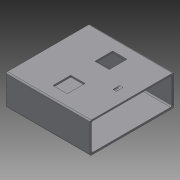
# Autodesk Inventor part: USB-Connector1
Saved by Autodesk Inventor 2015 (Build 190159000, 159)
## iProperties
Created: 2021-05-12
Part Number: USB-Connector1
Material: Generic
Document SubType Name: Modeling
Designer: bayua
Density: 1 g/cm^3
Appearance: Default
Author: bayua
Autodesk Inventor part; units mm, degrees
ref_plane "YZ Plane" through (0, 0, 0) normal (1, 0, 0) x (0, 1, 0)
ref_plane "XZ Plane" through (0, 0, 0) normal (0, 1, 0) x (-1, 0, 0)
ref_plane "XY Plane" through (0, 0, 0) normal (0, 0, 1) x (1, 0, 0)
sketch "Sketch2" plane through (0, 0, 0) normal (0, 0, 1) x (1, 0, 0)
  line L0 (-6.096, 6.096) -> (6.096, 6.096)
  line L1 (6.096, 6.096) -> (6.096, -6.096)
  line L2 (6.096, -6.096) -> (-6.096, -6.096)
  line L3 (-6.096, -6.096) -> (-6.096, 6.096)
  point P0 (0, 0)
  dimension "d4" = 12.192
  dimension "d5" = 12.192
  dimension "d6" = 6.096
  dimension "d7" = 6.096
  constraints: 8 end point, 2 parallel, 1 horizontal, 1 perpendicular
  measures "d4" distance of L0.end L1.end
  measures "d5" distance of L1.end L2.end
  measures "d6" distance from line of point (0, 0) L1
  measures "d7" distance from line of point (0, 0) L0
extrude "Extrusion1" add sketch "Sketch2" along normal mid plane 4.445
sketch "Sketch3" plane through (6.096, -6.096, 2.2225) normal (1, 0, 0) x (0, 0, -1)
  line L0 (0.254, 11.938) -> (4.191, 11.938)
  line L1 (4.191, 11.938) -> (4.191, 0.254)
  line L2 (4.191, 0.254) -> (0.254, 0.254)
  line L3 (0.254, 0.254) -> (0.254, 11.938)
  line L4 (0, 12.192) -> (0, 0) projected
  line L5 (4.445, 12.192) -> (0, 12.192) projected
  line L6 (4.445, 12.192) -> (4.445, 0) projected
  line L7 (0, 0) -> (4.445, 0) projected
  point P0 (2.2225, 6.096)
  dimension "d10" = 0.254
  dimension "d11" = 0.254
  dimension "d12" = 0.254
  dimension "d13" = 0.254
  constraints: 8 end point, 2 parallel, 1 horizontal, 1 perpendicular
  measures "d10" distance between parallel lines of L4 L3
  measures "d11" distance between parallel lines of L5 L0
  measures "d12" distance between parallel lines of L6 L1
  measures "d13" distance between parallel lines of L7 L2
extrude "Extrusion2" cut sketch "Sketch3" against normal through all contours L0 L1 L2 L3
sketch "Sketch4" plane through (0, 0, 2.2225) normal (0, 0, 1) x (1, 0, 0)
  line L0 (-1.016, 4.318) -> (1.016, 4.318)
  line L1 (1.016, 4.318) -> (1.016, 1.778)
  line L2 (1.016, 1.778) -> (-1.016, 1.778)
  line L3 (-1.016, 1.778) -> (-1.016, 4.318)
  line L4 (6.096, -6.096) -> (6.096, 6.096) projected
  line L5 (6.096, 6.096) -> (-6.096, 6.096) projected
  point P0 (0, 0)
  dimension "d16" = 5.08
  dimension "d17" = 1.778
  dimension "d18" = 2.54
  dimension "d19" = 2.032
  constraints: 8 end point, 2 parallel, 1 horizontal, 1 perpendicular
  measures "d16" distance between parallel lines of L4 L1
  measures "d17" distance between parallel lines of L5 L0
  measures "d18" distance of L0.end L1.end
  measures "d19" distance of L0.start L0.end
extrude "Extrusion3" cut sketch "Sketch4" against normal through all
mirror "Mirror1" about plane through (0, 0, 0) normal (0, 1, 0) of "Extrusion3"
sketch "Sketch5" plane through (0, 0, -2.2225) normal (0, 0, -1) x (-1, 0, 0)
  line L0 (-6.096, -6.096) -> (-6.096, 6.096) projected
  line L1 (6.096, 5.842) -> (6.096, -5.842) projected
  line L2 (-6.096, 0.0762) -> (6.096, 0.0762)
  line L3 (6.096, 0.0762) -> (6.096, -0.0762)
  line L4 (-6.096, -0.0762) -> (-6.096, 0.0762)
  line L5 (4.5615, -0.0961) -> (4.7095, -0.3103)
  line L6 (4.699, -0.3302) -> (4.318, -0.3302)
  line L7 (4.318, -0.3302) -> (4.318, -0.0762)
  line L8 (6.096, -0.0762) -> (4.572, -0.0762)
  arc A0 (4.572, -0.0762) -> (4.5615, -0.0961) centre (4.572, -0.0889) ccw
  arc A1 (4.699, -0.3302) -> (4.7095, -0.3103) centre (4.699, -0.3175) ccw
  line L9 (4.0745, -0.0961) -> (3.9265, -0.3103)
  line L10 (3.937, -0.3302) -> (4.318, -0.3302)
  arc A2 (4.0745, -0.0961) -> (4.064, -0.0762) centre (4.064, -0.0889) ccw
  arc A3 (3.9265, -0.3103) -> (3.937, -0.3302) centre (3.937, -0.3175) ccw
  line L11 (-4.5615, -0.0961) -> (-4.7095, -0.3103)
  line L12 (-4.699, -0.3302) -> (-4.318, -0.3302)
  arc A4 (-4.5615, -0.0961) -> (-4.572, -0.0762) centre (-4.572, -0.0889) ccw
  arc A5 (-4.7095, -0.3103) -> (-4.699, -0.3302) centre (-4.699, -0.3175) ccw
  arc A6 (-4.064, -0.0762) -> (-4.0745, -0.0961) centre (-4.064, -0.0889) ccw
  line L13 (-4.0745, -0.0961) -> (-3.9265, -0.3103)
  arc A7 (-3.937, -0.3302) -> (-3.9265, -0.3103) centre (-3.937, -0.3175) ccw
  line L14 (-3.937, -0.3302) -> (-4.318, -0.3302)
  line L15 (4.064, -0.0762) -> (-4.064, -0.0762)
  line L16 (-4.572, -0.0762) -> (-6.096, -0.0762)
  point P0 (0, 0)
  dimension "d22" = 0.0762
  dimension "d25" = 0.0762
  dimension "d26" = 0.254
  dimension "d27" = 0.0127
  dimension "d28" = 1.524
  dimension "d29" = 1.397
  dimension "d30" = 1.778
  constraints: 30 end point, 16 point on circle, 8 centre point, 6 symmetric about line, 4 tangent, 2 horizontal, 2 parallel, 2 perpendicular, 2 point on line, 1 equal radius, 2 other
  measures "d22" distance from line of point (0, 0) L2
  measures "d25" distance from line of point (0, 0) L8
  measures "d26" distance between parallel lines of L8 L6
  measures "d27" radius of A0
  measures "d28" distance from line of L1 A0.centre
  measures "d29" distance from line of L1 A1.centre
  measures "d30" distance from line of L1 L7.end
extrude "Extrusion4" add sketch "Sketch5" along normal blind 0.0032
sketch "Sketch6" plane through (0, 0, 2.2225) normal (0, 0, 1) x (1, 0, 0)
  line L0 (3.81, 0.508) -> (4.318, 0.508)
  line L1 (4.318, 0.508) -> (4.318, -0.508)
  line L2 (4.318, -0.508) -> (3.81, -0.508)
  line L3 (3.81, -0.508) -> (3.81, 0.508)
  line L4 (6.096, 6.096) -> (-6.096, 6.096) projected
  line L5 (6.096, -6.096) -> (6.096, 6.096) projected
  point P0 (0, 0)
  dimension "d33" = 5.588
  dimension "d34" = 1.778
  dimension "d35" = 0.508
  dimension "d36" = 1.016
  constraints: 8 end point, 2 parallel, 1 horizontal, 1 perpendicular
  measures "d33" distance between parallel lines of L4 L0
  measures "d34" distance between parallel lines of L5 L1
  measures "d35" distance of L0.start L0.end
  measures "d36" distance of L0.end L1.end
extrude "Extrusion5" cut sketch "Sketch6" against normal blind 0.127
fillet "Fillet1" radius 0.635 2 edges at (4.064, 0.508, 2.0955) (4.064, -0.508, 2.0955)
fillet "Fillet2" radius 0.0635 6 edges at (3.81, 0.3278, 2.1281) (3.81, -0.3278, 2.1281) (3.81, 0, 2.0955) (4.318, -0.3278, 2.1281) (4.318, 0.3278, 2.1281) (4.318, 0, 2.0955)
fillet "Fillet3" radius 0.1905 8 edges at (0, -6.096, 2.2225) (0, -5.842, 1.9685) (0, -5.842, -1.9685) (0, -6.096, -2.2225) (0, 5.842, -1.9685) (0, 6.096, -2.2225) (0, 6.096, 2.2225) (0, 5.842, 1.9685)
fillet "Fillet4" radius 0.0318 40 edges at (6.096, 5.7862, 1.9127) (6.096, 5.842, 0) (6.096, 5.7862, -1.9127) (6.096, 0, -1.9685) (6.096, -5.7862, -1.9127) (6.096, -5.842, 0) (6.096, -5.7862, 1.9127) (6.096, 0, 1.9685) (-6.096, -5.7862, 1.9127) (-6.096, -5.842, 0) (-6.096, -5.7862, -1.9127) (-6.096, 0, -1.9685) (-6.096, 5.7862, -1.9127) (-6.096, 5.842, 0) (-6.096, 5.7862, 1.9127) (-6.096, 0, 1.9685) (-1.016, -3.048, 1.9685) (-1.016, -3.048, 2.2225) (0, -4.318, 2.2225) (0, -4.318, 1.9685) (1.016, -3.048, 2.2225) (1.016, -3.048, 1.9685) (0, -1.778, 2.2225) (0, -1.778, 1.9685) (-1.016, -4.318, 2.0955) (1.016, -4.318, 2.0955) (1.016, -1.778, 2.0955) (-1.016, -1.778, 2.0955) (-1.016, 3.048, 1.9685) (-1.016, 3.048, 2.2225) (0, 4.318, 1.9685) (0, 4.318, 2.2225) (1.016, 3.048, 2.2225) (1.016, 3.048, 1.9685) (0, 1.778, 2.2225) (0, 1.778, 1.9685) (1.016, 1.778, 2.0955) (1.016, 4.318, 2.0955) (-1.016, 1.778, 2.0955) (-1.016, 4.318, 2.0955)
fillet "Fillet5" radius 0.0318 23 edges at (0, -4.318, -1.9685) (0, -4.318, -2.2225) (1.016, -3.048, -2.2225) (1.016, -3.048, -1.9685) (1.016, -4.318, -2.0955) (1.016, -1.778, -2.0955) (0, -1.778, -1.9685) (0, -1.778, -2.2225) (-1.016, -1.778, -2.0955) (-1.016, -3.048, -1.9685) (-1.016, -3.048, -2.2225) (0, 1.778, -1.9685) (0, 1.778, -2.2225) (-1.016, 1.778, -2.0955) (-1.016, 3.048, -1.9685) (-1.016, 3.048, -2.2225) (0, 4.318, -2.2225) (1.016, 3.048, -1.9685) (1.016, 3.048, -2.2225) (1.016, 1.778, -2.0955) (1.016, 4.318, -2.0955) (0, 4.318, -1.9685) (-1.016, 4.318, -2.0955)
equation "\"d5\" = d4"
equation "\"d7\" = d6"
equation "\"d11\" = d10"
equation "\"d12\" = d10"
equation "\"d13\" = d10"
body "Solid1"
